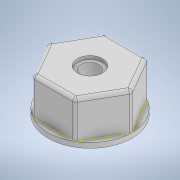
# Autodesk Inventor part: nut_simple
Saved by Autodesk Inventor 2020 (Build 240168000, 168)
## iProperties
Created: 2019-07-24
Part Number: nut_simple
Material: Generic
Document SubType Name: Modeling
Designer: erwin
Density: 1 g/cm^3
Appearance: Default
Author: erwin
Autodesk Inventor part; units mm, degrees
ref_plane "YZ Plane" through (0, 0, 0) normal (1, 0, 0) x (0, 1, 0)
ref_plane "XZ Plane" through (0, 0, 0) normal (0, 1, 0) x (-1, 0, 0)
ref_plane "XY Plane" through (0, 0, 0) normal (0, 0, 1) x (1, 0, 0)
sketch "Sketch1" plane through (0, 0, 0) normal (0, 1, 0) x (-1, 0, 0)
  circle A0 centre (0, 0) radius 25
  dimension "d0" = 50
  constraints: 1 centre point, 1 coincident
  measures "d0" diameter of A0
extrude "Extrusion1" add sketch "Sketch1" along normal blind 25
sketch "Sketch2" plane through (0, 25, 0) normal (0, 1, 0) x (1, 0, 0)
  circle A0 centre (0, 0) radius 25 projected
  constraints: 1 coincident
hole "Hole1" at (0, 25, 0) direction (0, -1, 0) diameter 9 end through all counterbore diameter 15 counterbore depth 2
sketch "Sketch3" plane through (0, 23, 0) normal (0, 1, 0) x (1, 0, 0)
  circle A0 centre (0, 0) radius 4.5 projected
  constraints: 1 coincident
hole "Hole2" at (0, 23, 0) direction (0, -1, 0) diameter 10.75 depth 17 tip angle 118
sketch "Sketch4" plane through (0, 25, 0) normal (0, 1, 0) x (1, 0, 0)
  circle A0 centre (0, 0) radius 25 projected
  line L0 (25, 0) -> (12.5, -21.6506)
  line L1 (12.5, -21.6506) -> (-12.5, -21.6506)
  line L2 (-12.5, -21.6506) -> (-25, 0)
  line L3 (-25, 0) -> (-12.5, 21.6506)
  line L4 (-12.5, 21.6506) -> (12.5, 21.6506)
  line L5 (12.5, 21.6506) -> (25, 0)
  point P0 (12.5, 21.6506)
  point P1 (12.5, 21.6506)
  point P2 (-25, 0)
  point P3 (-25, 0)
  point P4 (-12.5, -21.6506)
  point P5 (-12.5, -21.6506)
  constraints: 12 end point, 1 coincident, 15 other
extrude "Extrusion2" cut sketch "Sketch4" against normal blind 22 contours L5 A0 | A0 L0 | L4 A0 | A0 L1 | L3 A0 | A0 L2
sketch "Sketch6" plane through (0, 3, 0) normal (0, 1, 0) x (1, 0, 0)
  line L0 (12.5, -21.6506) -> (25, 0) projected
  line L1 (25, 0) -> (12.5, 21.6506) projected
  line L2 (12.5, 21.6506) -> (-12.5, 21.6506) projected
  line L3 (-12.5, 21.6506) -> (-25, 0) projected
  line L4 (-25, 0) -> (-12.5, -21.6506) projected
  line L5 (-12.5, -21.6506) -> (12.5, -21.6506) projected
  circle A0 centre (0, 0) radius 7.5 projected
fillet "Fillet1" radius 2 12 edges at (25, 14, 0) (12.5, 14, -21.6506) (-12.5, 14, -21.6506) (12.5, 14, 21.6506) (-25, 14, 0) (-12.5, 14, 21.6506) (-18.75, 25, 10.8253) (-18.75, 25, -10.8253) (0, 25, 21.6506) (18.75, 25, 10.8253) (18.75, 25, -10.8253) (0, 25, -21.6506)
body "Solid1"
